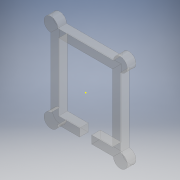
# Autodesk Inventor part: cubierta2
Saved by Autodesk Inventor 2016 (Build 200138000, 138)
## iProperties
Created: 2017-05-08
Part Number: cubierta2
Material: Generic
Document SubType Name: Modeling
Designer: rdiaz
Density: 1 g/cm^3
Appearance: Polycarbonate - Clear
Author: rdiaz
Autodesk Inventor part; units mm, degrees
ref_plane "YZ Plane" through (0, 0, 0) normal (1, 0, 0) x (0, 1, 0)
ref_plane "XZ Plane" through (0, 0, 0) normal (0, 1, 0) x (-1, 0, 0)
ref_plane "XY Plane" through (0, 0, 0) normal (0, 0, 1) x (1, 0, 0)
sketch "Sketch1" plane through (0, 0, 0) normal (0, 1, 0) x (-1, 0, 0)
  line L0 (19.5, 15.5) -> (-19.5, 15.5)
  line L1 (-19.5, -15.5) -> (19.5, -15.5)
  line L2 (19.5, -15.5) -> (19.5, 15.5)
  line L3 (24, -20) -> (-24, -20)
  line L4 (-24, 20) -> (24, 20)
  line L5 (24, 20) -> (24, -20)
  line L6 (-19.5, -3.5) -> (-24, -3.5)
  line L7 (-19.5, 3.5) -> (-24, 3.5)
  line L8 (-19.5, -3.5) -> (-19.5, -15.5)
  line L9 (-24, -20) -> (-24, -3.5)
  line L10 (-24, 3.5) -> (-24, 20)
  line L11 (-19.5, 3.5) -> (-19.5, 15.5)
  circle A0 centre (24, -20) radius 4
  circle A1 centre (24, 20) radius 4
  circle A2 centre (-24, 20) radius 4
  circle A3 centre (-24, -20) radius 4
  point P0 (0, 0)
  point P1 (0, -15.5)
  point P2 (19.5, 0)
  point P3 (0, 20)
  point P4 (24, 0)
  dimension "d0" = 39
  dimension "d1" = 31
  dimension "d2" = 4.5
  dimension "d25" = 4.5
  dimension "d27" = 4.5
  dimension "d28" = 16.5
  dimension "d29" = 8
  dimension "d30" = 8
  dimension "d31" = 8
  dimension "d32" = 8
  constraints: 24 end point, 5 parallel, 4 centre point, 4 coincident, 4 midpoint, 4 perpendicular, 3 equal length, 2 horizontal, 2 horizontal alignment, 2 vertical alignment, 1 vertical
  measures "d0" distance of L1.start L1.end
  measures "d1" distance of L1.end L0.start
  measures "d2" distance between parallel lines of L4 L0
  measures "d25" distance of L6.start L6.end
  measures "d27" distance between parallel lines of L5 L2
  measures "d28" distance of L3.end L6.end
  measures "d29" diameter of A0
  measures "d30" diameter of A1
  measures "d31" diameter of A2
  measures "d32" diameter of A3
extrude "Extrusion1" add sketch "Sketch1" along normal blind 5
sketch "Sketch2" plane through (0, 0, 0) normal (0, -1, 0) x (1, 0, 0)
  line L0 (-19.5, -15.5) -> (-19.5, 15.5) projected
  line L1 (-19.5, 15.5) -> (19.5, 15.5) projected
  line L2 (19.5, -15.5) -> (-19.5, -15.5) projected
  line L3 (24, -16) -> (24, -3.5) projected
  line L4 (20, 20) -> (-20, 20) projected
  line L5 (-24, 16) -> (-24, -16) projected
  line L6 (-20, -20) -> (20, -20) projected
  line L7 (19.5, -15.5) -> (-19.5, -15.5) construction
  line L8 (-40, 34) -> (40, 34) construction
  line L9 (40, 34) -> (40, -34) construction
  line L10 (40, -34) -> (-40, -34) construction
  line L11 (-40, -34) -> (-40, 34) construction
  line L12 (-40, 34) -> (-19.5, 15.5) construction
  line L13 (-40, -34) -> (-19.5, -15.5) construction
  line L14 (40, -34) -> (20, -15) construction
  line L15 (22, 18) -> (40, 34) construction
  line L16 (24, -3.5) -> (19.5, -3.5) projected
  line L17 (19.5, -3.5) -> (19.5, -15.5) projected
  line L18 (19.5, 3.5) -> (24, 3.5) projected
  line L19 (24, 3.5) -> (24, 16) projected
  line L20 (19.5, 15.5) -> (19.5, 3.5) projected
  arc A0 (-20, 20) -> (-24, 16) centre (-24, 20) ccw projected
  arc A1 (-24, -16) -> (-20, -20) centre (-24, -20) ccw projected
  arc A2 (20, -20) -> (24, -16) centre (24, -20) ccw projected
  arc A3 (24, 16) -> (20, 20) centre (24, 20) ccw projected
  point P0 (0, 0)
  point P1 (-40, 0)
  point P2 (0, 34)
  point P3 (-29.75, -24.75)
  point P4 (30, -24.5)
  point P5 (31, 26)
  point P6 (-29.75, 24.75)
  dimension "d14" = 54
  dimension "d15" = 64
  constraints: 16 end point, 6 midpoint, 2 parallel, 1 horizontal, 1 horizontal alignment, 1 perpendicular, 1 vertical alignment, 1 other
  measures "d14" distance between parallel lines of L4 L10
  measures "d15" distance between parallel lines of L11 L3
hole "Hole1" [suppressed]
sketch "Sketch3" plane through (0, 0, 0) normal (0, -1, 0) x (1, 0, 0)
  point P0 (0, 0)
body "Solid1"
